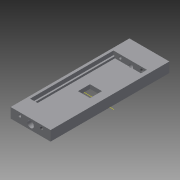
# Autodesk Inventor part: BottomSupportPlate
Saved by Autodesk Inventor 2015 SP1 (Build 190203100, 203)
## iProperties
Created: 2015-08-28
Part Number: BottomSupportPlate
Material: Generic
Document SubType Name: Modeling
Designer: I Rabey
Density: 1 g/cm^3
Appearance: Default
Author: I Rabey
Autodesk Inventor part; units mm, degrees
sketch "Sketch1" plane through (0, 0, 0) normal (0, 1, 0) x (-1, 0, 0)
  line L0 (-20, 59.5) -> (20, 59.5)
  line L1 (20, 59.5) -> (20, -59.5)
  line L2 (20, -59.5) -> (-20, -59.5)
  line L3 (-20, -59.5) -> (-20, 59.5)
  line L4 (-20, 59.5) -> (20, -59.5) construction
  line L5 (20, 59.5) -> (-20, -59.5) construction
  point P0 (0, 0)
  dimension "d0" = 40
  dimension "d1" = 119
  constraints: 12 end point, 2 midpoint, 2 parallel, 1 horizontal, 1 perpendicular
  measures "d0" distance of L1.end L2.end
  measures "d1" distance of L0.end L1.end
extrude "Extrusion1" add sketch "Sketch1" along normal blind 10
sketch "Sketch2" plane through (0, 10, 0) normal (0, 1, 0) x (1, 0, 0)
  line L0 (-16, -41) -> (-6, -41)
  line L1 (-6, -41) -> (-6, 41)
  line L2 (-6, 41) -> (-16, 41)
  line L3 (-16, 41) -> (-16, -41)
  line L4 (-16, -41) -> (-6, 41) construction
  line L5 (-6, -41) -> (-16, 41) construction
  line L6 (16, -41) -> (6, -41)
  line L7 (6, -41) -> (6, 41)
  line L8 (6, 41) -> (16, 41)
  line L9 (16, 41) -> (16, -41)
  line L10 (16, -41) -> (6, 41) construction
  line L11 (6, -41) -> (16, 41) construction
  line L12 (-6, -41) -> (6, -41)
  line L13 (6, -41) -> (6, 41)
  line L14 (6, 41) -> (-6, 41)
  line L15 (-6, 41) -> (-6, -41)
  line L16 (-6, -41) -> (6, 41) construction
  line L17 (6, -41) -> (-6, 41) construction
  point P0 (0, 0)
  point P1 (-11, 0)
  point P2 (11, 0)
  dimension "d4" = 10
  dimension "d5" = 82
  dimension "d6" = 11
  dimension "d7" = 0
  dimension "d8" = 10
  dimension "d9" = 82
  dimension "d10" = 11
  dimension "d21" = 12
  dimension "d22" = 82
  constraints: 36 end point, 6 midpoint, 6 parallel, 3 horizontal, 3 perpendicular
  measures "d4" distance of L2.end L1.end
  measures "d5" distance of L0.end L1.end
  measures "d6" distance of point (0, 0) point (-11, 0)
  measures "d7" vertical distance of point (0, 0) point (-11, 0)
  measures "d8" distance of L7.end L8.end
  measures "d9" distance of L6.end L7.end
  measures "d10" distance of point (0, 0) point (11, 0)
  measures "d21" distance of L14.end L13.end
  measures "d22" distance of L13.end L12.end
extrude "Extrusion3" cut sketch "Sketch2" against normal blind 6
sketch "Sketch3" plane through (0, 4, 0) normal (0, 1, 0) x (1, 0, 0)
  line L0 (-6, -6) -> (6, -6)
  line L1 (6, -6) -> (6, 6)
  line L2 (6, 6) -> (-6, 6)
  line L3 (-6, 6) -> (-6, -6)
  line L4 (-6, -6) -> (6, 6) construction
  line L5 (6, -6) -> (-6, 6) construction
  point P0 (0, 0)
  dimension "d35" = 12
  dimension "d36" = 12
  constraints: 12 end point, 2 midpoint, 2 parallel, 1 horizontal, 1 perpendicular
  measures "d35" distance of L2.end L1.end
  measures "d36" distance of L1.end L0.end
extrude "Extrusion4" cut sketch "Sketch3" against normal blind 6
ref_plane "Work Plane1" through (0, 4.5, 0) normal (0, 1, 0) x (-1, 0, 0)
ref_plane "Work Plane2" through (11, 0, 0) normal (1, 0, 0) x (0, 1, 0)
ref_plane "Work Plane3" through (-11, 0, 0) normal (1, 0, 0) x (0, 1, 0)
ref_plane "Work Plane7" through (-6, 4, -41) normal (0, 0, 1) x (1, 0, 0)
sketch "Sketch6" plane through (-6, 4, -41) normal (0, 0, 1) x (1, 0, 0)
  circle A0 centre (-5, 3) radius 1.5
  line L0 (0, 6) -> (0, 0) projected
  line L1 (-10, 6) -> (22, 6) projected
  line L2 (-10, 6) -> (-10, 0) projected
  point P0 (6, -4)
  point P1 (-9, 6)
  dimension "d42" = 3
  dimension "d44" = 3
  dimension "d112" = 5
  constraints: 1 centre point
  measures "d42" diameter of A0
  measures "d44" distance from line of L1 A0.centre
  measures "d112" distance from line of L2 A0.centre
ref_plane "Work Plane4" through (7, 4, -40) normal (0, 0, 1) x (1, 0, 0)
sketch "Sketch7" plane through (7, 4, -40) normal (0, 0, 1) x (1, 0, 0)
  circle A0 centre (4, 3) radius 1.5
  line L0 (0, 6) -> (8, 6) projected
  line L1 (9, 0) -> (9, 6) projected
  point P0 (-7, -4)
  dimension "d45" = 3
  dimension "d46" = 3
  dimension "d47" = 5
  constraints: 1 centre point
  measures "d45" diameter of A0
  measures "d46" distance from line of A0.centre L0
  measures "d47" distance from line of A0.centre L1
hole "Hole1" at (-11, 7, -41) direction (0, 0, -1) diameter 3 end through all
hole "Hole2" at (11, 7, -40) direction (0, 0, -1) diameter 3 end through all
ref_plane "Work Plane6" through (-6, 4, 41) normal (0, 0, -1) x (-1, 0, 0)
sketch "Sketch8" plane through (-6, 4, 41) normal (0, 0, -1) x (-1, 0, 0)
  circle A0 centre (5, 3) radius 1.5
  line L0 (-22, 6) -> (10, 6) projected
  line L1 (10, 0) -> (10, 6) projected
  point P0 (-6, -4)
  point P1 (0, 6)
  point P2 (9, 6)
  dimension "d62" = 3
  dimension "d63" = 3
  dimension "d64" = 5
  constraints: 1 centre point
  measures "d62" diameter of A0
  measures "d63" distance from line of A0.centre L0
  measures "d64" distance from line of L1 A0.centre
ref_plane "Work Plane5" through (7, 4, 40) normal (0, 0, -1) x (-1, 0, 0)
sketch "Sketch9" plane through (7, 4, 40) normal (0, 0, -1) x (-1, 0, 0)
  circle A0 centre (-4, 3) radius 1.5
  line L0 (-8, 6) -> (0, 6) projected
  line L1 (-9, 6) -> (-9, 0) projected
  point P0 (7, -4)
  dimension "d65" = 3
  dimension "d66" = 3
  dimension "d67" = 5
  constraints: 1 centre point
  measures "d65" diameter of A0
  measures "d66" distance from line of A0.centre L0
  measures "d67" distance from line of L1 A0.centre
hole "Hole3" at (-11, 7, 41) direction (0, 0, 1) diameter 3 end through all
hole "Hole4" at (11, 7, 40) direction (0, 0, 1) diameter 3 end through all
sketch "Sketch10" plane through (-20, 0, 59.5) normal (0, 0, 1) x (1, 0, 0)
  circle A0 centre (20, 5) radius 3.25
  line L0 (40, 0) -> (40, 10) projected
  point P0 (20, 0)
  dimension "d92" = 6.5
  dimension "d93" = 5
  dimension "d94" = 20
  constraints: 1 centre point
  measures "d92" diameter of A0
  measures "d93" distance of point (20, 0) A0.centre
  measures "d94" distance from line of L0 A0.centre
hole "Hole5" at (0, 5, 59.5) direction (0, 0, -1) diameter 6.5 depth 18.5
sketch "Sketch11" plane through (20, 0, -59.5) normal (0, 0, -1) x (-1, 0, 0)
  circle A0 centre (20, 5) radius 3.25
  line L0 (40, 0) -> (0, 0) projected
  line L1 (40, 0) -> (40, 10) projected
  point P0 (20, 0)
  dimension "d102" = 6.5
  dimension "d103" = 5
  dimension "d104" = 20
  constraints: 1 centre point
  measures "d102" diameter of A0
  measures "d103" distance from line of L0 A0.centre
  measures "d104" distance from line of L1 A0.centre
hole "Hole6" at (0, 5, -59.5) direction (0, 0, 1) diameter 6 depth 18 tip angle 118
sketch "Sketch12" plane through (0, 10, 0) normal (0, 1, 0) x (1, 0, 0)
  line L0 (-17.5, -41) -> (-16, -41)
  line L1 (-16, -41) -> (-16, 41)
  line L2 (-16, 41) -> (-17.5, 41)
  line L3 (-17.5, 41) -> (-17.5, -41)
  line L4 (-17.5, -41) -> (-16, 41) construction
  line L5 (-16, -41) -> (-17.5, 41) construction
  line L6 (-17.5, -42.5) -> (16, -42.5)
  line L7 (16, -42.5) -> (16, -41)
  line L8 (16, -41) -> (-17.5, -41)
  line L9 (-17.5, -41) -> (-17.5, -42.5)
  line L10 (-17.5, -42.5) -> (16, -41) construction
  line L11 (16, -42.5) -> (-17.5, -41) construction
  point P0 (0, 0)
  point P1 (-16.75, 0)
  point P2 (-0.75, -41.75)
  dimension "d113" = 1.5
  dimension "d114" = 82
  dimension "d115" = 16
  dimension "d116" = 33.5
  dimension "d117" = 1.5
  dimension "d118" = 0
  dimension "d128" = 0.75
  constraints: 24 end point, 4 midpoint, 4 parallel, 2 horizontal, 2 perpendicular
  measures "d113" distance of L2.end L1.end
  measures "d114" distance of L1.end L0.end
  measures "d115" distance from line of L1 point (0, 0)
  measures "d116" distance of L8.end L7.end
  measures "d117" distance of L7.end L6.end
  measures "d118" distance between parallel lines of L0 L8
  measures "d128" horizontal distance of point (0, 0) point (-0.75, -41.75)
extrude "Extrusion7" cut sketch "Sketch12" against normal blind 4
thread "Thread5" size "M3x0.5" class "6H" standard "ANSI Metric M Profile" full length
thread "Thread6" size "M3x0.5" class "6H" standard "ANSI Metric M Profile" full length
body "Solid1"
